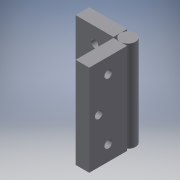
# Autodesk Inventor part: hinges (for assembly)
Saved by Autodesk Inventor 2016 (Build 200138000, 138)
## iProperties
Created: 2017-10-26
Part Number: hinges (for assembly)
Material: Generic
Document SubType Name: Modeling
Designer: student
Density: 1 g/cm^3
Appearance: Default
Author: student
Autodesk Inventor part; units mm, degrees
ref_plane "YZ Plane" through (0, 0, 0) normal (1, 0, 0) x (0, 1, 0)
ref_plane "XZ Plane" through (0, 0, 0) normal (0, 1, 0) x (-1, 0, 0)
ref_plane "XY Plane" through (0, 0, 0) normal (0, 0, 1) x (1, 0, 0)
sketch "Sketch1" plane through (0, 0, 0) normal (0, 0, 1) x (1, 0, 0)
  line L0 (-15.875, -38.1) -> (15.875, -38.1)
  line L1 (15.875, -38.1) -> (15.875, 38.1)
  line L2 (15.875, 38.1) -> (-15.875, 38.1)
  line L3 (-15.875, 38.1) -> (-15.875, -38.1)
  line L4 (-15.875, -38.1) -> (15.875, 38.1) construction
  line L5 (15.875, -38.1) -> (-15.875, 38.1) construction
  point P0 (0, 0)
  dimension "d0" = 76.2
  dimension "d1" = 31.75
  constraints: 12 end point, 2 midpoint, 2 parallel, 1 horizontal, 1 perpendicular
  measures "d0" distance of L2.end L0.start
  measures "d1" distance of L1.end L2.end
extrude "Extrusion1" add sketch "Sketch1" along normal blind 11.43
sketch "Sketch2" plane through (-15.875, 38.1, 0) normal (0, 1, 0) x (1, 0, 0)
  circle A0 centre (38.1, -5.715) radius 6.35
  line L0 (0, 0) -> (0, -11.43) projected
  line L1 (31.75, 0) -> (31.75, -11.43) projected
  line L2 (32.385, -43.815) -> (43.815, -43.815)
  line L3 (43.815, -43.815) -> (43.815, -12.065)
  line L4 (43.815, -12.065) -> (32.385, -12.065)
  line L5 (32.385, -12.065) -> (32.385, -43.815)
  line L6 (32.385, -43.815) -> (43.815, -12.065) construction
  line L7 (43.815, -43.815) -> (32.385, -12.065) construction
  point P0 (15.875, 0)
  point P1 (0, -5.715)
  point P2 (31.75, -5.715)
  point P3 (31.75, -5.715)
  point P4 (38.1, -27.94)
  point P5 (38.1, -12.065)
  point P6 (31.75, -5.715)
  point P7 (38.1, -27.94)
  dimension "d4" = 12.7
  dimension "d5" = 31.75
  dimension "d6" = 11.43
  constraints: 12 end point, 7 midpoint, 3 horizontal alignment, 2 coincident, 2 parallel, 2 vertical alignment, 1 horizontal, 1 perpendicular, 2 other
  measures "d5" distance of L2.end L3.end
  measures "d6" distance of L2.start L2.end
extrude "Extrusion2" add sketch "Sketch2" against normal blind 76.2
sketch "Sketch3" plane through (0, 0, 11.43) normal (0, 0, 1) x (1, 0, 0)
  circle A0 centre (-7.9375, 0) radius 3.175
  circle A1 centre (0, 25.4) radius 3.175
  circle A2 centre (0, -25.4) radius 3.175
  point P0 (0, 0)
  dimension "d9" = 6.35
  dimension "d10" = 7.9375
  dimension "d11" = 6.35
  dimension "d12" = 6.35
  dimension "d13" = 25.4
  dimension "d14" = 25.4
  constraints: 3 centre point
  measures "d9" diameter of A0
  measures "d10" distance of point (0, 0) A0.centre
  measures "d11" diameter of A1
  measures "d12" diameter of A2
  measures "d13" distance of point (0, 0) A2.centre
  measures "d14" distance of point (0, 0) A1.centre
sketch "Sketch4" plane through (16.51, 38.1, 12.065) normal (-1, 0, 0) x (0, 0, 1)
  circle A0 centre (23.8125, -38.1) radius 3.175
  circle A1 centre (15.875, -12.7) radius 3.175
  circle A2 centre (15.875, -63.5) radius 3.175
  line L0 (31.75, 0) -> (31.75, -76.2) projected
  line L1 (0, 0) -> (31.75, 0) projected
  line L2 (31.75, -76.2) -> (0, -76.2) projected
  line L3 (15.875, 0) -> (15.875, -76.2)
  line L4 (0, -76.2) -> (31.75, -76.2) projected
  line L5 (31.75, -38.1) -> (0.7842, -38.1)
  point P0 (-12.065, -38.1)
  dimension "d15" = 6.35
  dimension "d16" = 7.9375
  dimension "d17" = 25.4
  dimension "d18" = 25.4
  dimension "d19" = 6.35
  dimension "d20" = 6.35
  constraints: 4 end point, 3 centre point, 3 midpoint, 2 vertical alignment, 1 horizontal, 1 horizontal alignment, 1 perpendicular
  measures "d15" diameter of A0
  measures "d16" distance of L5.start A0.centre
  measures "d17" distance from line of L5 A1.centre
  measures "d18" distance from line of L5 A2.centre
  measures "d19" diameter of A1
  measures "d20" diameter of A2
hole "Hole1" at (0, 25.4, 11.43) at (-7.9375, 0, 11.43) at (0, -25.4, 11.43) direction (0, 0, -1) diameter 6.35 depth 25.4 tip angle 118
hole "Hole2" at (16.51, 0, 35.8775) at (16.51, -25.4, 27.94) at (16.51, 25.4, 27.94) direction (1, 0, 0) diameter 6.35 depth 25.4 tip angle 118
body "Solid1"
